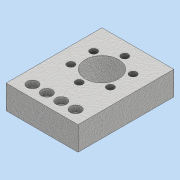
# Autodesk Inventor part: Obudowa nakrętki trapezowej fi 16 - oś Y
Saved by Autodesk Inventor 2018 (Build 220112000, 112)
## iProperties
Created: 2019-01-25
Part Number: Obudowa nakrętki trapezowej fi 16 - oś Y
Material: Ogólny
Document SubType Name: Modeling
Designer: Dawid
Density: 1 g/cm^3
Appearance: Aluminium odlewane
Author: Dawid
Autodesk Inventor part; units mm, degrees
ref_plane "YZ Plane" through (0, 0, 0) normal (1, 0, 0) x (0, 1, 0)
ref_plane "XZ Plane" through (0, 0, 0) normal (0, 1, 0) x (-1, 0, 0)
ref_plane "XY Plane" through (0, 0, 0) normal (0, 0, 1) x (1, 0, 0)
sketch "Szkic1" plane through (0, 0, 0) normal (0, 0, 1) x (1, 0, 0)
  line L0 (-30, -30) -> (30, -30)
  line L1 (30, -30) -> (30, 30)
  line L2 (30, 30) -> (-30, 30)
  line L3 (-30, 30) -> (-30, -30)
  line L4 (-30, -30) -> (30, 30) construction
  line L5 (30, -30) -> (-30, 30) construction
  point P0 (0, 0)
  dimension "d0" = 60
  dimension "d1" = 60
  constraints: 12 end point, 2 midpoint, 2 parallel, 1 horizontal, 1 perpendicular
  measures "d0" distance of L2.end L1.end
  measures "d1" distance of L1.end L0.end
extrude "Wyciągnięcie proste1" add sketch "Szkic1" along normal blind 35
sketch "Szkic2" plane through (0, 0, 35) normal (0, 0, 1) x (1, 0, 0)
  circle A0 centre (0, 0) radius 25
  dimension "d4" = 50
  constraints: 1 centre point, 1 coincident
  measures "d4" diameter of A0
extrude "Wyciągnięcie proste2" cut sketch "Szkic2" against normal blind 12
sketch "Szkic3" plane through (0, 0, 23) normal (0, 0, 1) x (1, 0, 0)
  circle A0 centre (0, 0) radius 14
  dimension "d7" = 28
  constraints: 1 centre point, 1 coincident
  measures "d7" diameter of A0
extrude "Wyciągnięcie proste3" cut sketch "Szkic3" against normal up to next
sketch "Szkic4" plane through (0, 0, 23) normal (0, 0, 1) x (1, 0, 0)
  circle A0 centre (0, 0) radius 19
  circle A1 centre (0, 19) radius 3
  circle A2 centre (-16.4545, 9.5) radius 3
  circle A3 centre (-16.4545, -9.5) radius 3
  circle A4 centre (0, -19) radius 3
  circle A5 centre (16.4545, -9.5) radius 3
  circle A6 centre (16.4545, 9.5) radius 3
  dimension "d10" = 38
  dimension "d11" = 6
  dimension "d14" = 360
  constraints: 6 centre point, 1 coincident, 1 vertical alignment, 15 other
  measures "d11" diameter of A1
sketch "Szkic13" plane through (0, 0, 35) normal (0, 0, 1) x (1, 0, 0)
  circle A0 centre (0, 0) radius 25 projected
  line L0 (-30, -30) -> (30, -30) projected
  line L1 (30, -30) -> (30, 30) projected
  line L2 (30, 30) -> (-30, 30) projected
  line L3 (-30, 30) -> (-30, -30) projected
extrude "Wyciągnięcie proste10" cut sketch "Szkic13" against normal up to surface (12 mm away)
extrude "Wyciągnięcie proste11" cut sketch "Szkic4" against normal up to next contours A6 A0 | A0 A6 | A5 A0 | A0 A5 | A1 A0 | A0 A1 | A4 A0 | A0 A4 | A2 A0 | A0 A2 | A3 A0 | A0 A3
thread "Gwint7" size "M6x1" class "6H" standard "ANSI Metric M Profile" full length
thread "Gwint8" size "M6x1" class "6H" standard "ANSI Metric M Profile" full length
thread "Gwint9" size "M6x1" class "6H" standard "ANSI Metric M Profile" full length
thread "Gwint10" size "M6x1" class "6H" standard "ANSI Metric M Profile" full length
thread "Gwint11" size "M6x1" class "6H" standard "ANSI Metric M Profile" full length
thread "Gwint12" size "M6x1" class "6H" standard "ANSI Metric M Profile" full length
sketch "Szkic14" plane through (0, 0, 0) normal (0, 0, -1) x (-1, 0, 0)
  circle A0 centre (0, 0) radius 14 projected
  line L0 (30, -30) -> (-30, -30) projected
  line L1 (30, 30) -> (30, -30) projected
  line L2 (-30, 30) -> (30, 30) projected
  line L3 (-30, -30) -> (-30, 30) projected
extrude "Wyciągnięcie proste12" cut sketch "Szkic14" against normal blind 3
sketch "Szkic16" plane through (-30, -30, 23) normal (0, -1, 0) x (1, 0, 0)
  line L0 (0, -20) -> (60, -20) projected
  line L1 (60, -20) -> (60, 0) projected
  line L2 (60, 0) -> (0, 0) projected
  line L3 (0, -20) -> (0, 0) projected
  point P0 (30, -23)
extrude "Wyciągnięcie proste14" add sketch "Szkic16" along normal blind 20
sketch "Szkic17" plane through (0, 0, 23) normal (0, 0, 1) x (1, 0, 0)
  circle A0 centre (16.4545, 9.5) radius 3 projected
  circle A1 centre (0, -19) radius 3 projected
  circle A2 centre (-16.4545, 9.5) radius 3 projected
  circle A3 centre (0, 19) radius 3 projected
  circle A4 centre (-16.4545, -9.5) radius 3 projected
  circle A5 centre (16.4545, -9.5) radius 3 projected
  line L0 (30, 30) -> (30, -50) projected
  line L1 (-30, 30) -> (30, 30) projected
  line L2 (-30, -50) -> (-30, 30) projected
  line L3 (30, -50) -> (-30, -50) projected
  circle A6 centre (0, 0) radius 14 projected
  line L4 (-30, -50) -> (-30, -40)
  line L5 (-30, 30) -> (-30, -50) projected
  line L6 (-30, -40) -> (30, -40)
  line L7 (30, -50) -> (30, 30) projected
  line L8 (-30, -40) -> (-18, -40)
  line L9 (-18, -40) -> (-6, -40)
  line L10 (-6, -40) -> (6, -40)
  line L11 (6, -40) -> (18, -40)
  circle A7 centre (-18, -40) radius 2.5
  circle A8 centre (-6, -40) radius 2.5
  circle A9 centre (6, -40) radius 2.5
  circle A10 centre (18, -40) radius 2.5
  dimension "d100" = 10
  dimension "d101" = 12
  dimension "d102" = 12
  dimension "d103" = 12
  dimension "d104" = 12
  dimension "d105" = 5
  dimension "d106" = 5
  dimension "d107" = 5
  dimension "d108" = 5
  constraints: 12 end point, 6 point on line, 4 centre point, 4 coincident, 1 perpendicular
  measures "d100" distance of L2.start L4.end
  measures "d101" distance of L4.end L8.end
  measures "d102" distance of L8.end L9.end
  measures "d103" distance of L9.end L10.end
  measures "d104" distance of L10.end L11.end
  measures "d105" diameter of A7
  measures "d106" diameter of A8
  measures "d107" diameter of A9
  measures "d108" diameter of A10
hole "Otwór1" at (-18, -40, 23) at (-6, -40, 23) at (6, -40, 23) at (18, -40, 23) direction (0, 0, -1) diameter 5 end through all counterbore diameter 9 counterbore depth 5
